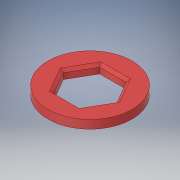
# Autodesk Inventor part: spacerForEndV08
Saved by Autodesk Inventor 2019.4 (Build 234330000, 330)
## iProperties
Created: 2019-02-25
Part Number: spacerForEndV08
Material: PC/ABS Plastic
Document SubType Name: Modeling
Designer: steele
Density: 0.357273 g/cm^3
Appearance: Smooth - Red
holeForString: 0.200 in
stringDiameter: 0.120 in
clearanceForString: 0.080 in
hexShaftDiameter: 0.500 in
clearanceForHexShaft: 0.045 in
hexDiameter: 0.545 in
supportChannels: 0.150 in
spoolInteriorDiameter: 1.500 in
spoolInteriroRadius: 0.750 in
spoolExteriorDiameter: 3.500 in
spoolExteriorRadius: 1.750 in
spoolFiletRadius: 0.075 in
holeCenter: 0.575 in
hexHoleChamfer: 0.063 in
stringHoleCenterFromHexShaft: 0.373 in
textCircleDiameter: 2.625 in
textHeight: 0.240 in
textDepth: 0.050 in
stringHoleChamfer: 0.188 in
spoolTotalHeight: 3.000 in
spaceHeight: 0.250 in
spacerDiameter: 0.950 in
spoolHeightWithoutSpacer: 2.750 in
Author: steele
Autodesk Inventor part; units mm, degrees
ref_plane "YZ Plane" through (0, 0, 0) normal (1, 0, 0) x (0, 1, 0)
ref_plane "XZ Plane" through (0, 0, 0) normal (0, 1, 0) x (-1, 0, 0)
ref_plane "XY Plane" through (0, 0, 0) normal (0, 0, 1) x (1, 0, 0)
sketch "Sketch9" plane through (0, 0, 0) normal (0, 1, 0) x (-1, 0, 0)
  circle A0 centre (0, 0) radius 12.6365
  dimension "d53" = 25.273
  constraints: 1 centre point, 1 coincident
  measures "d53" diameter of A0
extrude "Extrusion6" add sketch "Sketch9" along normal mid plane 2.54
sketch "Sketch15" plane through (0, 1.27, 0) normal (0, 1, 0) x (1, 0, 0)
  line L0 (7.9923, 0) -> (3.9961, -6.9215)
  line L1 (3.9961, -6.9215) -> (-3.9961, -6.9215)
  line L2 (-3.9961, -6.9215) -> (-7.9923, 0)
  line L3 (-7.9923, 0) -> (-3.9961, 6.9215)
  line L4 (-3.9961, 6.9215) -> (3.9961, 6.9215)
  line L5 (3.9961, 6.9215) -> (7.9923, 0)
  point P0 (0, 0)
  point P1 (0, 0)
  dimension "d82" = 13.843
  constraints: 12 end point, 1 coincident, 13 other
  measures "d82" distance between parallel lines of L1 L4
extrude "Extrusion11" cut sketch "Sketch15" against normal through all
chamfer "Chamfer7" distance 0.7937 angle 45 6 edges at (-5.9942, 1.27, -3.4607) (-5.9942, 1.27, 3.4608) (0, 1.27, 6.9215) (5.9942, 1.27, 3.4607) (5.9942, 1.27, -3.4608) (0, 1.27, -6.9215)
equation "\"d82\" = hexDiameter"
equation "\"holeForString\" = stringDiameter + clearanceForString"
equation "\"stringDiameter\" = 3.048"
equation "\"clearanceForString\" = 2.032"
equation "\"spoolHeightWithoutSpacer\" = 69.85"
equation "\"hexShaftDiameter\" = 12.7"
equation "\"clearanceForHexShaft\" = 1.143"
equation "\"hexDiameter\" = hexShaftDiameter + clearanceForHexShaft"
equation "\"supportChannels\" = 3.81"
equation "\"spoolInteriorDiameter\" = 38.1"
equation "\"spoolInteriroRadius\" = 0.5 * spoolInteriorDiameter"
equation "\"spoolExteriorDiameter\" = 88.9"
equation "\"spoolExteriorRadius\" = 0.5 * spoolExteriorDiameter"
equation "\"spoolFiletRadius\" = 0.5 * supportChannels"
equation "\"holeCenter\" = 0.25 * spoolHeightWithoutSpacer - 0.75 * supportChannels"
equation "\"hexHoleChamfer\" = 1.5875"
equation "\"stringHoleCenterFromHexShaft\" = 0.5 * hexDiameter + 0.5 * holeForString"
equation "\"textCircleDiameter\" = 0.75 * spoolExteriorDiameter"
equation "\"textHeight\" = 6.096"
equation "\"textDepth\" = 1.27"
equation "\"stringHoleChamfer\" = 4.7625"
equation "\"spoolTotalHeight\" = 76.2"
equation "\"spaceHeight\" = spoolTotalHeight - spoolHeightWithoutSpacer"
equation "\"spacerDiameter\" = 24.13"
body "Solid1"
body "Solid2"
